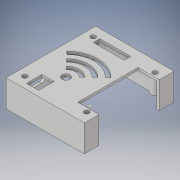
# Autodesk Inventor part: Box2_Top
Saved by Autodesk Inventor 2017 (Build 210142000, 142)
## iProperties
Created: 2017-11-18
Part Number: Box2_Top
Material: Generic
Document SubType Name: Modeling
Designer: Arthur Bondar
Density: 1 g/cm^3
Appearance: Default
Author: Arthur Bondar
Autodesk Inventor part; units mm, degrees
ref_plane "YZ Plane" through (0, 0, 0) normal (1, 0, 0) x (0, 1, 0)
ref_plane "XZ Plane" through (0, 0, 0) normal (0, 1, 0) x (-1, 0, 0)
ref_plane "XY Plane" through (0, 0, 0) normal (0, 0, 1) x (1, 0, 0)
sketch "Sketch1" plane through (0, 0, 0) normal (0, 1, 0) x (-1, 0, 0)
  point P0 (0, 0)
sketch "Sketch2" plane through (0, 0, 0) normal (0, 1, 0) x (-1, 0, 0)
  line L0 (-24, 27.5) -> (24, 27.5)
  line L1 (24, 27.5) -> (24, -27.5)
  line L2 (24, -27.5) -> (-24, -27.5)
  line L3 (-24, -27.5) -> (-24, 27.5)
  line L4 (22.5, 26) -> (-22.5, 26)
  line L5 (-22.5, 26) -> (-22.5, -26)
  line L6 (-22.5, -26) -> (22.5, -26)
  line L7 (22.5, -26) -> (22.5, 26)
  dimension "d1" = 55
  constraints: 16 end point, 4 parallel, 2 horizontal, 2 perpendicular
  measures "d1" distance of L0.end L1.end
extrude "Extrusion1" add sketch "Sketch2" along normal blind 6
sketch "Sketch3" plane through (0, 6, 0) normal (0, 1, 0) x (1, 0, 0)
  circle A0 centre (19, -21) radius 2.5
  circle A1 centre (-19, -21) radius 2.5
  circle A2 centre (-19, 21) radius 2.5
  circle A3 centre (19, 21) radius 2.5
  circle A4 centre (-19, -21) radius 1.5
  circle A5 centre (-19, 21) radius 1.5
  circle A6 centre (19, 21) radius 1.5
  circle A7 centre (19, -21) radius 1.5
  line L0 (-22.5, -26) -> (22.5, -26)
  line L1 (22.5, -26) -> (22.5, 26)
  line L2 (22.5, 26) -> (-22.5, 26)
  line L3 (-22.5, 26) -> (-22.5, -26)
  line L4 (-24, -27.5) -> (24, -27.5)
  line L5 (24, -27.5) -> (24, 27.5)
  line L6 (24, 27.5) -> (-24, 27.5)
  line L7 (-24, 27.5) -> (-24, -27.5)
  dimension "d16" = 3
  dimension "d17" = 3
  dimension "d18" = 3
  constraints: 16 end point, 8 centre point, 4 coincident, 4 parallel, 2 horizontal, 2 perpendicular
  measures "d16" diameter of A4
  measures "d17" diameter of A6
  measures "d18" diameter of A7
extrude "Extrusion2" add sketch "Sketch3" along normal blind 9
sketch "Sketch4" plane through (24, 0, 27.5) normal (1, 0, 0) x (0, 0, -1)
  line L0 (9, 6) -> (9, 15) projected
  line L1 (9, 15) -> (46, 15)
  line L2 (55, 0) -> (0, 0) projected
  line L3 (46, 6) -> (46, 15)
  line L4 (46, 15) -> (9, 15)
  line L5 (9, 15) -> (9, 6)
  line L6 (9, 0) -> (46, 0)
  line L7 (46, 0) -> (46, 15)
  line L8 (46, 15) -> (9, 15)
  line L9 (9, 15) -> (9, 0)
  point P0 (27.5, 0)
  constraints: 16 end point, 3 parallel, 2 point on line, 1 horizontal, 1 perpendicular
extrude "Extrusion3" cut sketch "Sketch4" against normal up to surface (1.5 mm away)
sketch "Sketch5" plane through (0, 15, 0) normal (0, 1, 0) x (1, 0, 0)
  line L0 (-24, -27.5) -> (24, -27.5) projected
  line L1 (-24, 27.5) -> (-24, -27.5) projected
  line L2 (24, -27.5) -> (-24, -27.5)
  line L3 (-24, -27.5) -> (-24, 27.5)
  line L4 (-24, 27.5) -> (24, 27.5)
  line L5 (22.5, -18.5) -> (24, -18.5) projected
  line L6 (24, -18.5) -> (11, -18.5)
  line L7 (24, 18.5) -> (24, 27.5) projected
  line L8 (24, 18.5) -> (11, 18.5)
  line L9 (11, 18.5) -> (11, -18.5)
  line L10 (24, 27.5) -> (24, 18.5)
  line L11 (24, -18.5) -> (24, -27.5)
  circle A0 centre (-19, -21) radius 1.5 projected
  circle A1 centre (-19, -21) radius 1.5
  circle A2 centre (-19, 21) radius 1.5 projected
  circle A3 centre (-19, 21) radius 1.5
  circle A4 centre (19, 21) radius 1.5 projected
  circle A5 centre (19, 21) radius 1.5
  circle A6 centre (19, -21) radius 1.5 projected
  circle A7 centre (19, -21) radius 1.5
  point P0 (0, 0)
  constraints: 16 end point, 4 centre point, 4 coincident, 3 parallel, 2 horizontal, 2 perpendicular, 1 collinear
extrude "Extrusion4" add sketch "Sketch5" along normal blind 1.5
sketch "Sketch6" plane through (-24, 0, -27.5) normal (-1, 0, 0) x (0, 0, 1)
  line L0 (55, 0) -> (55, 16.5) projected
  line L1 (41.3229, 12.25) -> (34.9286, 12.25)
  line L2 (34.9286, 4.25) -> (41.3229, 4.25)
  arc A0 (41.3229, 4.25) -> (41.3229, 12.25) centre (41.3229, 8.25) ccw
  arc A1 (34.9286, 12.25) -> (34.9286, 4.25) centre (34.9286, 8.25) ccw
  point P0 (27.5, 0)
  constraints: 4 end point, 4 point on circle, 4 tangent, 2 centre point, 1 parallel
extrude "Extrusion5" cut sketch "Sketch6" against normal up to surface (1.5 mm away)
sketch "Sketch7" plane through (0, 16.5, 0) normal (0, 1, 0) x (1, 0, 0)
  circle A0 centre (-19, 21) radius 1.5 projected
  line L0 (3, 18) -> (-16, 18)
  line L1 (-16, 18) -> (-16, 22)
  line L2 (-16, 22) -> (3, 22)
  line L3 (3, 22) -> (3, 18)
  point P0 (0, 0)
  dimension "d37" = 19
  dimension "d38" = 4
  constraints: 8 end point, 2 parallel, 1 horizontal, 1 perpendicular
  measures "d37" distance of L1.end L2.end
  measures "d38" distance of L0.end L1.end
extrude "Extrusion6" cut sketch "Sketch7" against normal through all contours L0 L1 L2 L3
sketch "Sketch8" plane through (0, 16.5, 0) normal (0, 1, 0) x (1, 0, 0)
  line L0 (-14.75, -24.25) -> (-7.25, -24.25)
  line L1 (-7.25, -24.25) -> (-7.25, -14.75)
  line L2 (-7.25, -14.75) -> (-14.75, -14.75)
  line L3 (-14.75, -14.75) -> (-14.75, -24.25)
  point P0 (0, 0)
  dimension "d44" = 7.5
  dimension "d45" = 9.5
  constraints: 8 end point, 2 parallel, 1 horizontal, 1 perpendicular
  measures "d44" distance of L2.end L1.end
  measures "d45" distance of L1.end L0.end
extrude "Extrusion7" cut sketch "Sketch8" against normal through all
sketch "Sketch9" plane through (0, 16.5, 0) normal (0, 1, 0) x (1, 0, 0)
  circle A0 centre (-5.9739, -8.7344) radius 2.43
  arc A1 (-1.887, -4.8042) -> (-9.9041, -4.6475) centre (-5.9739, -8.7344) ccw
  arc A2 (-0.1355, -3.1199) -> (-11.5884, -2.8959) centre (-5.9739, -8.7344) ccw
  arc A3 (2.1999, -0.874) -> (-13.8342, -0.5606) centre (-5.9739, -8.7344) ccw
  arc A4 (3.9514, 0.8103) -> (-15.5186, 1.1909) centre (-5.9739, -8.7344) ccw
  arc A5 (6.2868, 3.0561) -> (-17.7644, 3.5263) centre (-5.9739, -8.7344) ccw
  arc A6 (8.0389, 4.741) -> (-19.3203, 5.4014) centre (-5.9739, -8.7344) ccw
  line L0 (-19.3203, 5.4014) -> (-19.4487, 5.2778)
  line L1 (-19.4487, 5.2778) -> (-19.3445, 5.1695)
  line L2 (-17.7644, 3.5263) -> (-19.3445, 5.1695)
  line L3 (-13.8342, -0.5606) -> (-15.5186, 1.1909)
  line L4 (-9.9041, -4.6475) -> (-11.5884, -2.8959)
  line L5 (-1.887, -4.8042) -> (-0.1355, -3.1199)
  line L6 (2.1999, -0.874) -> (3.9514, 0.8103)
  line L7 (6.2868, 3.0561) -> (8.0389, 4.741)
  point P0 (0, 0)
  dimension "d48" = 4.86
  constraints: 16 end point, 12 point on circle, 7 centre point, 6 coincident, 1 perpendicular
  measures "d48" diameter of A0
extrude "Extrusion8" cut sketch "Sketch9" against normal through all
body "Solid1"
